Autodesk Inventor part; units mm, degrees
(part 2 of 2)
sketch "Sketch17" plane through (0, 0, 1) normal (0, 0, 1) x (1, 0, 0)
  line L0 (-216.6958, 8.1128) -> (-213.7696, 8.1128) projected
  line L1 (-217.0851, 5.7213) -> (-216.6958, 8.1128) projected
  line L2 (-216.0327, 5.5715) -> (-217.0851, 5.7213) projected
  spline S0 degree 2 poles (-215.7632, 5.7983) (-215.883, 5.7384) (-216.0327, 5.5715) knots 0 0 0 1 1 1 projected
  spline S1 degree 2 poles (-215.4166, 5.8881) (-215.5963, 5.8881) (-215.7632, 5.7983) knots 0 0 0 1 1 1 projected
  spline S2 degree 2 poles (-214.8006, 5.1223) (-214.8006, 5.5202) (-215.1386, 5.8881) (-215.4166, 5.8881) knots 0 0 0 0.5 1 1 1 projected
  spline S3 degree 2 poles (-215.391, 4.3437) (-215.1343, 4.3437) (-214.8006, 4.733) (-214.8006, 5.1223) knots 0 0 0 0.5 1 1 1 projected
  spline S4 degree 2 poles (-215.9985, 4.9555) (-215.9514, 4.656) (-215.622, 4.3437) (-215.391, 4.3437) knots 0 0 0 0.5 1 1 1 projected
  line L3 (-217.2477, 4.8186) -> (-215.9985, 4.9555) projected
  spline S5 degree 2 poles (-215.3781, 3.5908) (-215.8188, 3.5908) (-216.4434, 3.7576) (-216.8841, 4.087) (-217.1579, 4.5063) (-217.2477, 4.8186) knots 0 0 0 0.25 0.5 0.75 1 1 1 projected
  spline S6 degree 2 poles (-213.5556, 5.2336) (-213.5556, 4.8058) (-213.9835, 4.01) (-214.7664, 3.5908) (-215.3781, 3.5908) knots 0 0 0 0.333333 0.666667 1 1 1 projected
  spline S7 degree 2 poles (-215.0487, 6.6539) (-214.3856, 6.6539) (-213.5556, 5.8453) (-213.5556, 5.2336) knots 0 0 0 0.5 1 1 1 projected
  spline S8 degree 2 poles (-215.853, 6.4614) (-215.6477, 6.5555) (-215.2455, 6.6539) (-215.0487, 6.6539) knots 0 0 0 0.5 1 1 1 projected
  line L4 (-215.7503, 7.1288) -> (-215.853, 6.4614) projected
  line L5 (-213.7696, 7.1288) -> (-215.7503, 7.1288) projected
  line L6 (-213.7696, 8.1128) -> (-213.7696, 7.1288) projected
  line L7 (-213.2947, 8.1128) -> (-211.8572, 8.1128) projected
  line L8 (-211.6134, 3.6678) -> (-213.2947, 8.1128) projected
  line L9 (-210.1246, 3.6678) -> (-211.6134, 3.6678) projected
  line L10 (-208.4732, 8.1128) -> (-210.1246, 3.6678) projected
  line L11 (-209.8679, 8.1128) -> (-208.4732, 8.1128) projected
  line L12 (-210.8519, 4.9127) -> (-209.8679, 8.1128) projected
  line L13 (-211.8572, 8.1128) -> (-210.8519, 4.9127) projected
  line L14 (-185.1975, 8.1128) -> (-185.1975, 3.5908) projected
  line L15 (-186.2199, 8.1128) -> (-185.1975, 8.1128) projected
  spline S9 degree 2 poles (-187.743, 6.9234) (-187.1141, 7.1245) (-186.4167, 7.6935) (-186.2199, 8.1128) knots 0 0 0 0.5 1 1 1 projected
  line L16 (-187.743, 5.9095) -> (-187.743, 6.9234) projected
  spline S10 degree 2 poles (-186.4467, 6.5555) (-186.7504, 6.3245) (-187.3151, 6.0421) (-187.743, 5.9095) knots 0 0 0 0.5 1 1 1 projected
  line L17 (-186.4467, 3.5908) -> (-186.4467, 6.5555) projected
  line L18 (-185.1975, 3.5908) -> (-186.4467, 3.5908) projected
  line L19 (-180.2391, 3.5908) -> (-183.944, 3.5908) projected
  line L20 (-180.2391, 4.5961) -> (-180.2391, 3.5908) projected
  line L21 (-182.1685, 4.5961) -> (-180.2391, 4.5961) projected
  spline S11 degree 2 poles (-181.3728, 5.225) (-181.745, 4.9683) (-181.9974, 4.763) (-182.1685, 4.5961) knots 0 0 0 0.5 1 1 1 projected
  spline S12 degree 2 poles (-180.269, 6.8165) (-180.269, 6.4101) (-180.7439, 5.6699) (-181.3728, 5.225) knots 0 0 0 0.5 1 1 1 projected
  spline S13 degree 2 poles (-182.0616, 8.1128) (-181.4113, 8.1128) (-180.684, 7.8133) (-180.269, 7.2015) (-180.269, 6.8165) knots 0 0 0 0.333333 0.666667 1 1 1 projected
  spline S14 degree 2 poles (-183.8541, 6.6924) (-183.7814, 7.2144) (-183.3921, 7.8005) (-182.6862, 8.1128) (-182.0616, 8.1128) knots 0 0 0 0.333333 0.666667 1 1 1 projected
  line L22 (-182.6177, 6.594) -> (-183.8541, 6.6924) projected
  spline S15 degree 2 poles (-182.0273, 7.2657) (-182.2669, 7.2657) (-182.5664, 6.9705) (-182.6177, 6.594) knots 0 0 0 0.5 1 1 1 projected
  spline S16 degree 2 poles (-181.5011, 6.7737) (-181.5011, 6.9791) (-181.8006, 7.2657) (-182.0273, 7.2657) knots 0 0 0 0.5 1 1 1 projected
  spline S17 degree 2 poles (-182.3439, 5.7641) (-181.8049, 6.1662) (-181.5011, 6.5855) (-181.5011, 6.7737) knots 0 0 0 0.5 1 1 1 projected
  spline S18 degree 2 poles (-183.944, 3.5908) (-183.8798, 4.1384) (-183.2338, 5.1052) (-182.3439, 5.7641) knots 0 0 0 0.5 1 1 1 projected
  line L23 (-179.9482, 8.0358) -> (-178.5107, 8.0358) projected
  line L24 (-178.2669, 3.5908) -> (-179.9482, 8.0358) projected
  line L25 (-176.7781, 3.5908) -> (-178.2669, 3.5908) projected
  line L26 (-175.1267, 8.0358) -> (-176.7781, 3.5908) projected
  line L27 (-176.5214, 8.0358) -> (-175.1267, 8.0358) projected
  line L28 (-177.5053, 4.8357) -> (-176.5214, 8.0358) projected
  line L29 (-178.5107, 8.0358) -> (-177.5053, 4.8357) projected
  point P0 (0, 0)
  constraints: 19 other
extrude "Extrusion14" add sketch "Sketch17" along normal blind 1 separate body
sketch "Sketch18" plane through (0, 0, 2) normal (0, 0, 1) x (1, 0, 0)
  line L0 (-180.2391, 4.5961) -> (-180.2391, 3.5908) projected
  line L1 (-180.2391, 3.5908) -> (-183.944, 3.5908) projected
  line L2 (-182.6177, 6.594) -> (-183.8541, 6.6924) projected
  line L3 (-182.1685, 4.5961) -> (-180.2391, 4.5961) projected
  line L4 (-211.6134, 3.6678) -> (-213.2947, 8.1128) projected
  line L5 (-213.2947, 8.1128) -> (-211.8572, 8.1128) projected
  line L6 (-211.8572, 8.1128) -> (-210.8519, 4.9127) projected
  line L7 (-210.8519, 4.9127) -> (-209.8679, 8.1128) projected
  line L8 (-209.8679, 8.1128) -> (-208.4732, 8.1128) projected
  line L9 (-208.4732, 8.1128) -> (-210.1246, 3.6678) projected
  line L10 (-210.1246, 3.6678) -> (-211.6134, 3.6678) projected
  line L11 (-217.0851, 5.7213) -> (-216.6958, 8.1128) projected
  line L12 (-216.6958, 8.1128) -> (-213.7696, 8.1128) projected
  line L13 (-213.7696, 8.1128) -> (-213.7696, 7.1288) projected
  line L14 (-213.7696, 7.1288) -> (-215.7503, 7.1288) projected
  line L15 (-215.7503, 7.1288) -> (-215.853, 6.4614) projected
  line L16 (-217.2477, 4.8186) -> (-215.9985, 4.9555) projected
  line L17 (-216.0327, 5.5715) -> (-217.0851, 5.7213) projected
  line L18 (-186.2199, 8.1128) -> (-185.1975, 8.1128) projected
  line L19 (-185.1975, 8.1128) -> (-185.1975, 3.5908) projected
  line L20 (-185.1975, 3.5908) -> (-186.4467, 3.5908) projected
  line L21 (-186.4467, 3.5908) -> (-186.4467, 6.5555) projected
  line L22 (-187.743, 5.9095) -> (-187.743, 6.9234) projected
  line L23 (-178.2669, 3.5908) -> (-179.9482, 8.0358) projected
  line L24 (-179.9482, 8.0358) -> (-178.5107, 8.0358) projected
  line L25 (-178.5107, 8.0358) -> (-177.5053, 4.8357) projected
  line L26 (-177.5053, 4.8357) -> (-176.5214, 8.0358) projected
  line L27 (-176.5214, 8.0358) -> (-175.1267, 8.0358) projected
  line L28 (-175.1267, 8.0358) -> (-176.7781, 3.5908) projected
  line L29 (-176.7781, 3.5908) -> (-178.2669, 3.5908) projected
  circle A0 centre (-212.9631, 17.5895) radius 6.2905 projected
  circle A1 centre (-212.9631, 55.6895) radius 6.2905 projected
  circle A2 centre (-181.6894, 36.6395) radius 6.2905 projected
  circle A3 centre (-181.6894, 17.5895) radius 6.2905 projected
  circle A4 centre (-212.9631, 36.6395) radius 6.2905 projected
  circle A5 centre (-181.6894, 55.6895) radius 6.2905 projected
  line L30 (-191.2299, 65.23) -> (-191.2299, 6.049) projected
  line L31 (-191.2299, 6.049) -> (-193.2299, 6.049) projected
  line L32 (-193.2299, 6.049) -> (-193.2299, 67.23) projected
  line L33 (-193.2299, 67.23) -> (-170.1489, 67.23) projected
  line L34 (-170.1489, 67.23) -> (-170.1489, 6.049) projected
  line L35 (-170.1489, 6.049) -> (-172.1489, 6.049) projected
  line L36 (-172.1489, 6.049) -> (-172.1489, 65.23) projected
  line L37 (-172.1489, 65.23) -> (-191.2299, 65.23) projected
  line L38 (-224.5036, 6.049) -> (-224.5036, 67.23) projected
  line L39 (-224.5036, 67.23) -> (-201.4226, 67.23) projected
  line L40 (-201.4226, 67.23) -> (-201.4226, 6.049) projected
  line L41 (-201.4226, 6.049) -> (-203.4226, 6.049) projected
  line L42 (-203.4226, 6.049) -> (-203.4226, 65.23) projected
  line L43 (-203.4226, 65.23) -> (-222.5036, 65.23) projected
  line L44 (-222.5036, 65.23) -> (-222.5036, 6.049) projected
  line L45 (-222.5036, 6.049) -> (-224.5036, 6.049) projected
  line L46 (-228.6, 69.85) -> (-228.6, 0) projected
  line L47 (-228.6, 0) -> (0, 0) projected
  line L48 (0, 0) -> (0, 69.85) projected
  line L49 (0, 69.85) -> (-228.6, 69.85) projected
  line L50 (-142.24, 40.005) -> (-166.0525, 40.005) projected
  line L51 (-166.0525, 40.005) -> (-166.0525, 62.23) projected
  line L52 (-166.0525, 62.23) -> (-142.24, 62.23) projected
  line L53 (-142.24, 62.23) -> (-142.24, 40.005) projected
  line L54 (-142.24, 6.35) -> (-166.0525, 6.35) projected
  line L55 (-166.0525, 6.35) -> (-166.0525, 28.575) projected
  line L56 (-166.0525, 28.575) -> (-142.24, 28.575) projected
  line L57 (-142.24, 28.575) -> (-142.24, 6.35) projected
  line L58 (-108.2675, 40.005) -> (-132.08, 40.005) projected
  line L59 (-132.08, 40.005) -> (-132.08, 62.23) projected
  line L60 (-132.08, 62.23) -> (-108.2675, 62.23) projected
  line L61 (-108.2675, 62.23) -> (-108.2675, 40.005) projected
  line L62 (-74.295, 40.005) -> (-98.1075, 40.005) projected
  line L63 (-98.1075, 40.005) -> (-98.1075, 62.23) projected
  line L64 (-98.1075, 62.23) -> (-74.295, 62.23) projected
  line L65 (-74.295, 62.23) -> (-74.295, 40.005) projected
  line L66 (-40.3225, 40.005) -> (-64.135, 40.005) projected
  line L67 (-64.135, 40.005) -> (-64.135, 62.23) projected
  line L68 (-64.135, 62.23) -> (-40.3225, 62.23) projected
  line L69 (-40.3225, 62.23) -> (-40.3225, 40.005) projected
  line L70 (-6.35, 40.005) -> (-30.1625, 40.005) projected
  line L71 (-30.1625, 40.005) -> (-30.1625, 62.23) projected
  line L72 (-30.1625, 62.23) -> (-6.35, 62.23) projected
  line L73 (-6.35, 62.23) -> (-6.35, 40.005) projected
  line L74 (-108.2675, 6.35) -> (-132.08, 6.35) projected
  line L75 (-132.08, 6.35) -> (-132.08, 28.575) projected
  line L76 (-132.08, 28.575) -> (-108.2675, 28.575) projected
  line L77 (-108.2675, 28.575) -> (-108.2675, 6.35) projected
  line L78 (-74.295, 6.35) -> (-98.1075, 6.35) projected
  line L79 (-98.1075, 6.35) -> (-98.1075, 28.575) projected
  line L80 (-98.1075, 28.575) -> (-74.295, 28.575) projected
  line L81 (-74.295, 28.575) -> (-74.295, 6.35) projected
  line L82 (-40.3225, 6.35) -> (-64.135, 6.35) projected
  line L83 (-64.135, 6.35) -> (-64.135, 28.575) projected
  line L84 (-64.135, 28.575) -> (-40.3225, 28.575) projected
  line L85 (-40.3225, 28.575) -> (-40.3225, 6.35) projected
  line L86 (-6.35, 6.35) -> (-30.1625, 6.35) projected
  line L87 (-30.1625, 6.35) -> (-30.1625, 28.575) projected
  line L88 (-30.1625, 28.575) -> (-6.35, 28.575) projected
  line L89 (-6.35, 28.575) -> (-6.35, 6.35) projected
  circle A6 centre (-212.9631, 55.6895) radius 6.5405
  circle A7 centre (-212.9631, 36.6395) radius 6.5405
  circle A8 centre (-212.9631, 17.5895) radius 6.5405
  circle A9 centre (-181.6894, 17.5895) radius 6.5405
  circle A10 centre (-181.6894, 36.6395) radius 6.5405
  circle A11 centre (-181.6894, 55.6895) radius 6.5405
  dimension "d126" = 0.25
  dimension "d127" = 0.25
  dimension "d128" = 0.25
  dimension "d129" = 0.25
  dimension "d130" = 0.25
  dimension "d131" = 0.25
  constraints: 6 centre point, 19 other
  measures "d126" radial gap between concentric circles of A1 A6
  measures "d127" radial gap between concentric circles of A4 A7
  measures "d128" radial gap between concentric circles of A0 A8
  measures "d129" radial gap between concentric circles of A3 A9
  measures "d130" radial gap between concentric circles of A2 A10
  measures "d131" radial gap between concentric circles of A5 A11
extrude "Extrusion15" cut sketch "Sketch18" against normal up to surface (4 mm away) contours A6 | A7 | A8 | A9 | A10 | A11 bodies 1
body "Solid1"
body "Solid3"
body "Solid5"
